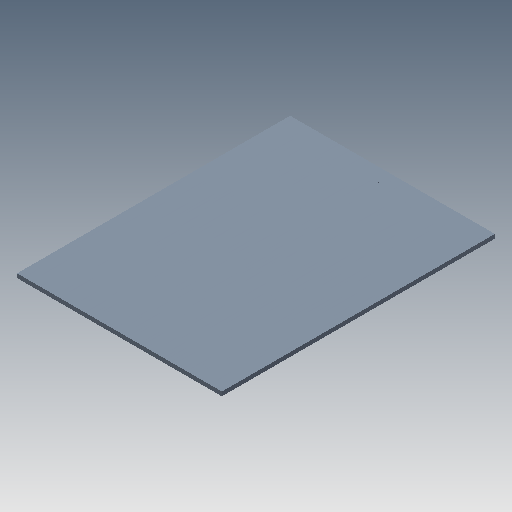
# Autodesk Inventor part: Instrumentation Panel Board
Saved by Autodesk Inventor 2020 (Build 240152000, 152)
## iProperties
Created: 2009-08-11
Part Number: Instrumentation Panel Board
Material: Polyaryletherketone Resin
Document SubType Name: Modeling
Designer: Demir Ali
Mass: 14849.6 g
Surface Area: 15528.8 cm^2
Volume: 11249.7 cm^3
Density: 1.32 g/cm^3
Appearance: Steel Blue
Description: Instrumentation Panel Board
Stock Number: NA
Author: Demir Ali
Title: Manufactured Part
Revision Number: A
Autodesk Inventor part; units mm, degrees
ref_plane "YZ Plane" through (0, 0, 0) normal (1, 0, 0) x (0, 1, 0)
ref_plane "XZ Plane" through (0, 0, 0) normal (0, 1, 0) x (-1, 0, 0)
ref_plane "XY Plane" through (0, 0, 0) normal (0, 0, 1) x (1, 0, 0)
derived "Instrumentation_Frame_SK.ipt"
sketch "Board_SK" plane through (-300, -20, 0) normal (0, -1, 0) x (1, 0, 0)
  line L0 (600, 1800) -> (0, 1800)
  line L1 (0, 0) -> (0, 1800)
  line L2 (0, 0) -> (600, 0)
  line L3 (600, 0) -> (600, 1800)
  line L4 (-75, 1875) -> (675, 1875)
  line L5 (675, 1875) -> (675, 875)
  line L6 (675, 875) -> (-75, 875)
  line L7 (-75, 875) -> (-75, 1875)
  point P0 (300, 0)
  point P1 (300, 1800)
  point P2 (300, 1875)
extrude "Extrusion1" add sketch "Board_SK" along normal blind 15 contours L3 L6 L1 L0 | L0 L1 L6 L7 L4 L5 L3
sketch "Sketch2" plane through (-375, -35, 1875) normal (0, -1, 0) x (1, 0, 0)
  line L0 (0, 0) -> (750, 0) projected
  circle A0 centre (225, -175) radius 50
  line L1 (0, 0) -> (750, 0) projected
  line L2 (375, 0) -> (375, -1000) construction
  line L3 (750, -1000) -> (0, -1000) projected
  line L4 (225, -175) -> (225, -450) construction
  line L5 (750, -1000) -> (0, -1000) projected
  line L6 (375, -950) -> (375, -675) construction
  circle A1 centre (375, -675) radius 50
  point P0 (375, -1875)
  dimension "d3" = 150
  dimension "d4" = 175
  dimension "d5" = 100
  dimension "d6" = 275
  dimension "d20" = 0
  dimension "d21" = 500
  constraints: 6 end point, 2 centre point, 2 midpoint, 2 perpendicular, 1 coincident, 1 equal radius, 1 parallel
  measures "d3" distance from line of L2 L4.start
  measures "d4" distance from line of L0 L4.start
  measures "d5" diameter of A0
  measures "d6" distance of L4.start L4.end
  measures "d20" distance from line of L2 A1.centre
  measures "d21" vertical distance of A1.centre L4.start
hole "Hole1" at (-150, -35, 1425) direction (0, 1, 0) diameter 3 end through all
pattern_linear "Rectangular Pattern1" count 2 spacing 300 along (1, 0, 0) of "Hole1"
hole "Hole2" at (0, -35, 925) direction (0, 1, 0) diameter 3 end through all
equation "\"d16\" = 2 * d3"
body "Solid1"
